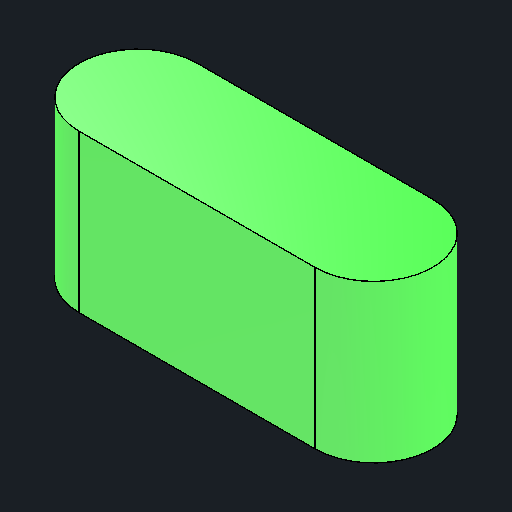
# Autodesk Inventor part: Status Indicator
Saved by Autodesk Inventor 2026.2 (Build 302298000, 298)
## iProperties
Created: 2026-05-29
Part Number: Status Indicator
Material: Polycarbonate, Clear
Document SubType Name: Modeling
Designer: JoshuaEah
Density: 1.2 g/cm^3
Appearance: LED - Green On
Author: JoshuaEah
Autodesk Inventor part; units mm, degrees
ref_plane "YZ Plane" through (0, 0, 0) normal (1, 0, 0) x (0, 1, 0)
ref_plane "XZ Plane" through (0, 0, 0) normal (0, 1, 0) x (-1, 0, 0)
ref_plane "XY Plane" through (0, 0, 0) normal (0, 0, 1) x (1, 0, 0)
sketch "Sketch1" plane through (0, 0, 0) normal (0, 1, 0) x (-1, 0, 0)
  line L0 (1.5, 0) -> (-1.5, 0) construction
  line L1 (1.5, 0.75) -> (-1.5, 0.75)
  line L2 (-1.5, -0.75) -> (1.5, -0.75)
  arc A0 (1.5, -0.75) -> (1.5, 0.75) centre (1.5, 0) ccw
  arc A1 (-1.5, 0.75) -> (-1.5, -0.75) centre (-1.5, 0) ccw
  point P0 (0, 0)
  dimension "d0" = 1.5
  dimension "d1" = 1.5
  constraints: 8 end point, 4 point on circle, 4 tangent, 2 centre point, 1 horizontal, 1 midpoint, 1 parallel
  measures "d0" distance of point (0, 0) L0.end
  measures "d1" diameter of A1
extrude "Extrusion1" add sketch "Sketch1" along normal blind 2
body "Solid1"
